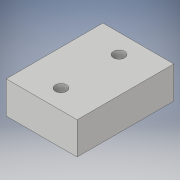
# Autodesk Inventor part: Detector fil - base
Saved by Autodesk Inventor 2019 (Build 230136000, 136)
## iProperties
Created: 2018-09-19
Part Number: Detector fil - base
Material: Genérico
Document SubType Name: Modeling
Designer: Albert Garangou Culebras
Density: 1 g/cm^3
Appearance: Valor por defecto
Author: Albert Garangou Culebras
Autodesk Inventor part; units mm, degrees
ref_plane "YZ Plane" through (0, 0, 0) normal (1, 0, 0) x (0, 1, 0)
ref_plane "XZ Plane" through (0, 0, 0) normal (0, 1, 0) x (-1, 0, 0)
ref_plane "XY Plane" through (0, 0, 0) normal (0, 0, 1) x (1, 0, 0)
sketch "Boceto1" plane through (0, 0, 0) normal (0, 1, 0) x (-1, 0, 0)
  line L0 (0, 0) -> (-22, 0)
  line L1 (-22, 0) -> (-22, -30)
  line L2 (-22, -30) -> (0, -30)
  line L3 (0, -30) -> (0, 0)
  line L4 (-11, 0) -> (-11, -6)
  line L5 (-11, -30) -> (-11, -24)
  circle A0 centre (-11, -6) radius 1.75
  circle A1 centre (-11, -24) radius 1.75
  dimension "d0" = 22
  dimension "d1" = 30
  dimension "d2" = 6
  dimension "d3" = 6
  dimension "d4" = 3.5
  dimension "d5" = 3.5
  constraints: 12 end point, 2 centre point, 2 coincident, 2 midpoint, 2 parallel, 2 perpendicular, 1 horizontal, 1 vertical
  measures "d0" distance of L2.end L1.end
  measures "d1" distance of L1.end L0.end
  measures "d2" distance of L4.start L4.end
  measures "d3" distance of L5.start L5.end
  measures "d4" diameter of A0
  measures "d5" diameter of A1
extrude "Extrusión1" add sketch "Boceto1" along normal blind 10
